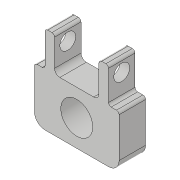
# Autodesk Inventor part: Needle Bearing Mount v2
Saved by Autodesk Inventor 2018.3 (Build 223284000, 284)
## iProperties
Created: 2019-03-08
Part Number: Needle Bearing Mount v2
Material: Generic
Document SubType Name: Modeling
Designer: aye06091
Mass: 23.767 g
Surface Area: 78.4556 cm^2
Volume: 23.767 cm^3
Density: 1 g/cm^3
Appearance: Default
Author: aye06091
Autodesk Inventor part; units mm, degrees
ref_plane "YZ Plane" through (0, 0, 0) normal (1, 0, 0) x (0, 1, 0)
ref_plane "XZ Plane" through (0, 0, 0) normal (0, 1, 0) x (-1, 0, 0)
ref_plane "XY Plane" through (0, 0, 0) normal (0, 0, 1) x (1, 0, 0)
sketch "Sketch1" plane through (0, 0, 0) normal (0, 0, 1) x (1, 0, 0)
  line L0 (0, 0) -> (50.8, 0)
  line L1 (50.8, 0) -> (50.8, -31.75)
  line L2 (50.8, -31.75) -> (0, -31.75)
  line L3 (0, -31.75) -> (0, 0)
  line L4 (6.35, 0) -> (12.065, 0)
  line L5 (12.065, 0) -> (12.065, 20.955)
  line L6 (12.065, 20.955) -> (6.35, 20.955)
  line L7 (6.35, 20.955) -> (6.35, 0)
  line L8 (38.735, 0) -> (44.45, 0)
  line L9 (44.45, 0) -> (44.45, 20.955)
  line L10 (44.45, 20.955) -> (38.735, 20.955)
  line L11 (38.735, 20.955) -> (38.735, 0)
  dimension "d1" = 31.75
  dimension "d4" = 5.715
  dimension "d5" = 5.715
  dimension "d21" = 20.955
  dimension "d29" = 6.35
  dimension "d30" = 6.35
  dimension "d32" = 50.8
  constraints: 24 end point, 6 parallel, 3 horizontal, 3 perpendicular, 3 point on line
  measures "d1" distance of L2.end L0.start
  measures "d4" distance between parallel lines of L9 L11
  measures "d5" distance of L5.end L6.end
  measures "d21" distance of L6.end L4.start
  measures "d29" distance between parallel lines of L3 L7
  measures "d30" distance from line of L0.end L9
  measures "d32" distance between parallel lines of L1 L3
extrude "Extrusion1" add sketch "Sketch1" against normal blind 15.875
sketch "Sketch2" plane through (0, 0, 0) normal (0, 0, 1) x (1, 0, 0)
  circle A0 centre (25.4, -15.875) radius 9.5885
  line L0 (50.8, -31.75) -> (0, -31.75) projected
  line L1 (0, 0) -> (0, -31.75)
  dimension "d10" = 19.177
  dimension "d24" = 15.875
  dimension "d31" = 25.4
  constraints: 2 end point, 1 centre point, 1 vertical
  measures "d10" diameter of A0
  measures "d24" distance from line of L0 A0.centre
  measures "d31" distance from line of L1 A0.centre
extrude "Extrusion2" cut sketch "Sketch2" against normal through all
sketch "Sketch3" plane through (44.45, 0, 0) normal (1, 0, 0) x (0, 0, -1)
  line L0 (0, 20.955) -> (15.875, 20.955) projected
  circle A0 centre (7.9375, 13.335) radius 4.7625
  dimension "d13" = 9.525
  dimension "d15" = 7.62
  constraints: 1 centre point
  measures "d13" diameter of A0
  measures "d15" distance from line of L0 A0.centre
extrude "Extrusion3" cut sketch "Sketch3" against normal up to next
fillet "Fillet2" radius 6.35 2 edges at (50.8, -31.75, -7.9375) (0, -31.75, -7.9375)
fillet "Fillet4" radius 1.5875 8 edges at (50.8, 0, -7.9375) (44.45, 0, -7.9375) (44.45, 20.955, -7.9375) (38.735, 20.955, -7.9375) (12.065, 20.955, -7.9375) (6.35, 20.955, -7.9375) (0, 0, -7.9375) (6.35, 0, -7.9375)
fillet "Fillet5" radius 3.175 2 edges at (12.065, 0, -7.9375) (38.735, 0, -7.9375)
sketch "Sketch4" plane through (12.065, 19.3675, 0) normal (1, 0, 0) x (0, 0, -1)
  circle A0 centre (7.9375, -6.0325) radius 4.7625 projected
  circle A1 centre (7.9375, -6.0325) radius 4.7625
  point P0 (0, -19.3675)
  dimension "d26" = 9.525
  constraints: 1 centre point, 1 coincident
  measures "d26" diameter of A1
extrude "Extrusion4" cut sketch "Sketch4" against normal through all
body "Solid1"
